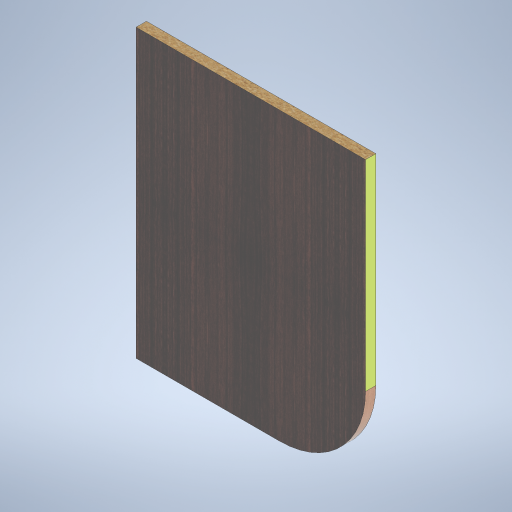
# Autodesk Inventor part: Example
Saved by Autodesk Inventor 2024 (Build 280153000, 153)
## iProperties
Created: 2022-05-27
Part Number: Example
Material: LMDF
Document SubType Name: Modeling
Designer: OlgerdA
Density: 0.8 g/cm^3
Appearance: LMDF Fill
Mass: 2810.47 g
Surface Area: 4215.84 cm^2
Volume: 3513.09 cm^3
Length: 501.0
Width: 401.0
Thickness: 18.0
Material Code: LMDF
Color Code: B02
Right Edge: B02
Back Edge: PNTB 02
Item Type: Part
Item_length: 501.0
Item_width: 401.0
Item_thickness: 18.0
Author: OlgerdA
Autodesk Inventor part; units mm, degrees
ref_plane "YZ Plane" through (0, 0, 0) normal (1, 0, 0) x (0, 1, 0)
ref_plane "XZ Plane" through (0, 0, 0) normal (0, 1, 0) x (-1, 0, 0)
ref_plane "XY Plane" through (0, 0, 0) normal (0, 0, 1) x (1, 0, 0)
sketch "Sketch1" plane through (0, 0, 0) normal (0, 0, 1) x (1, 0, 0)
  line L0 (0, 0) -> (400, 0)
  line L1 (400, 0) -> (400, 500)
  line L2 (400, 500) -> (0, 500)
  line L3 (0, 500) -> (0, 0)
  dimension "d0" = 400
  dimension "d1" = 500
  constraints: 8 end point, 2 parallel, 1 horizontal, 1 perpendicular
  measures "d0" distance of L2.end L1.end
  measures "d1" distance of L1.end L0.end
extrude "Extrusion1" add sketch "Sketch1" along normal blind 18
fillet "Fillet1" radius 150 1 edges at (400, 0, 9)
body "Solid1"
